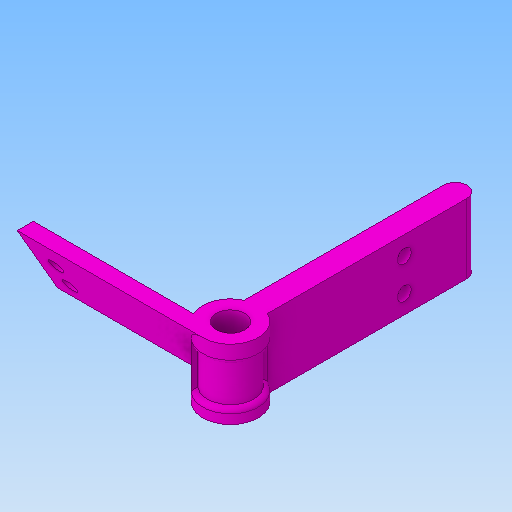
# Autodesk Inventor part: Pancake_Switch Lever
Saved by Autodesk Inventor 2018.1 (Build 221171000, 171)
## iProperties
Created: 2019-03-01
Part Number: Pancake_Switch Lever
Material: ABS Plastic
Document SubType Name: Modeling
Designer: James
Density: 1.06 g/cm^3
Appearance: Magenta
Mass: 6.48807 g
Surface Area: 43.5194 cm^2
Volume: 6.12082 cm^3
Author: James
Autodesk Inventor part; units mm, degrees
ref_plane "XZ Plane" through (0, 0, 0) normal (0, 1, 0) x (-1, 0, 0)
ref_plane "XY Plane" through (0, 0, 0) normal (0, 0, 1) x (1, 0, 0)
sketch "Sketch1" plane through (0, 0, 0) normal (0, 1, 0) x (-1, 0, 0)
  circle A0 centre (0, 0) radius 6
  line L0 (-2.5, 0) -> (2.5, 0)
  line L1 (2.5, 0) -> (2.5, -51)
  line L2 (2.5, -51) -> (-2.5, -51)
  line L3 (-2.5, -51) -> (-2.5, 0)
  dimension "d0" = 12
  dimension "d1" = 5
  dimension "d3" = 51
  constraints: 8 end point, 2 coincident, 2 parallel, 1 centre point, 1 horizontal, 1 midpoint, 1 perpendicular
  measures "d0" diameter of A0
  measures "d1" distance of L0.start L0.end
  measures "d3" distance of L0.end L1.end
extrude "Extrusion1" add sketch "Sketch1" along normal blind 15
ref_plane "Work Plane1" through (0, 0, 0) normal (1, 0, 0) x (0, 1, 0)
sketch "Sketch2" plane through (0, 0, 0) normal (1, 0, 0) x (0, 1, 0)
  line L0 (15, -5.4544) -> (0, -5.4544) projected
  line L1 (0, -5.4544) -> (0, -5.4544) projected
  line L2 (0, -5.4544) -> (15, -5.4544) projected
  line L3 (15, 2.5359) -> (15, 6)
  line L4 (15, 6) -> (0, -2.6603)
  line L5 (0, 6) -> (0, -5.4544) projected
  line L6 (0, -2.6603) -> (0, -6.1244)
  line L7 (0, -6.1244) -> (15, 2.5359)
  line L8 (0, 6) -> (15, 6) projected
  line L9 (15, -5.4544) -> (15, 6) projected
  point P0 (0, 0)
  point P1 (10.5616, 3.716)
  dimension "d7" = 3
  dimension "d9" = 60
  dimension "d19" = 0
  constraints: 8 end point, 2 point on line, 1 collinear, 1 parallel, 1 vertical, 1 other
  measures "d7" distance between parallel lines of L4 L7
  measures "d9" angle of L3 L7
extrude "Extrusion2" add sketch "Sketch2" against normal blind 40 contours L7 L6 L0 | L0 L5 L4 L3 L7
full round fillet "Fillet1" first side at (-2.5, 10, -20.8596) centre faces at (-0.8333, 5, -51) second side at (2.5, 5, -35.8181)
sketch "Sketch3" plane through (0, 15, 0) normal (0, 1, 0) x (1, 0, 0)
  point P0 (0, 0)
  point P1 (0, 0)
  constraints: 1 coincident
hole "Hole1" at (0, 15, 0) direction (0, -1, 0) diameter 6.2 end through all
chamfer "Chamfer1" distance 0.5 angle 45 1 edges at (0, 0, -3.1)
sketch "Sketch4" plane through (-2.5, 1.1605, -5.4544) normal (-1, 0, 0) x (0, 0, 1)
  line L0 (-43.0456, 13.8395) -> (0, 13.8395) projected
  line L1 (5.4544, -4.1605) -> (5.4544, 16.8395) projected
  line L2 (0, 13.8395) -> (-43.0456, 13.8395) projected
  point P0 (5.4544, -1.1605)
  point P1 (-29.5456, 9.8395)
  point P2 (-29.5456, 2.8395)
  dimension "d23" = 4
  dimension "d24" = 35
  dimension "d32" = 7
  constraints: 1 vertical alignment
  measures "d23" distance from line of L0 point (-29.546, 9.84)
  measures "d24" distance from line of L1 point (-29.546, 9.84)
  measures "d32" distance of point (-29.546, 9.84) point (-29.546, 2.84)
hole "Hole2" at (-2.5, 11, -35) at (-2.5, 4, -35) direction (1, 0, 0) diameter 3 end through all
ref_plane "Work Plane3" through (2.5, 0, -5.4544) normal (0.9090593, 0, 0.4166667) x (0, 1, 0)
sketch "Sketch7" plane through (2.5, 0, -5.4544) normal (0.9090593, 0, 0.4166667) x (0, 1, 0)
  ellipse E0 centre (4.6077, 6) end of major axis (-5.7303, 0.319) minor radius 2.2025 (15, 11.4544) -> (0, 5.8225) ccw projected
  line L0 (0, 0) -> (0, 5.8225) projected
  line L1 (0, 0) -> (15, 0) projected
  line L2 (15, 11.4544) -> (15, 0) projected
  line L3 (11, 0) -> (3, 0)
  line L4 (3, 0) -> (3, 1)
  line L5 (3, 1) -> (11, 1)
  line L6 (11, 1) -> (11, 0)
  line L7 (-3.5552, 6) -> (18.1287, 6) projected
  point P0 (0, 6)
  dimension "d52" = 1
  dimension "d53" = 4
  dimension "d54" = 3
  constraints: 8 end point, 2 parallel, 1 horizontal, 1 perpendicular, 1 point on line, 1 other
  measures "d52" distance of L5.end L3.start
  measures "d53" distance between parallel lines of L2 L6
  measures "d54" distance between parallel lines of L0 L4
revolve "Revolution2" cut sketch "Sketch7" angle 195 about axis through (0, -10, 0) along (0, -1, 0) contours L1 L4 L5 L6
fillet "Fillet2" radius 1 2 edges at (5.0814, 3, 3.1905) (5.0814, 11, 3.1905)
sketch "Sketch8" plane through (-2.5, 0, -6.1244) normal (0, 0.5, -0.8660254) x (-1, 0, 0)
  line L0 (2.9378, 17.3205) -> (37.5, 17.3205) projected
  line L1 (37.5, 17.3205) -> (37.5, 0) projected
  point P0 (-2.5, 3.0622)
  point P1 (32.5, 12.3205)
  point P2 (32.5, 6.3205)
  dimension "d57" = 6
  dimension "d58" = 5
  dimension "d59" = 5
  constraints: 1 vertical alignment
  measures "d57" distance of point (32.5, 6.321) point (32.5, 12.321)
  measures "d58" distance from line of L0 point (32.5, 12.321)
  measures "d59" distance from line of L1 point (32.5, 12.321)
hole "Hole3" at (-35, 10.6699, 0.0359) at (-35, 5.4737, -2.9641) direction (0, -0.5, 0.8660254) diameter 3 end through all
body "Solid1"
